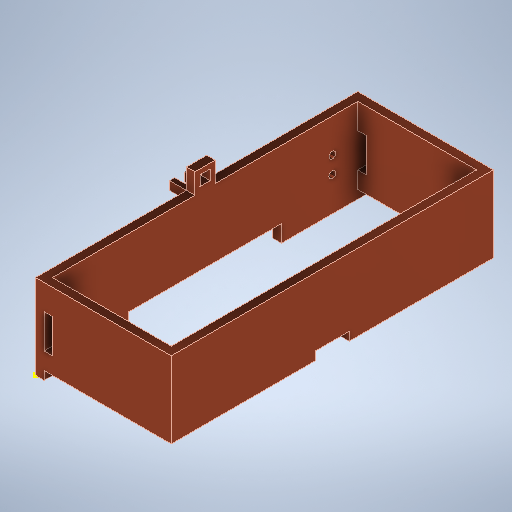
# Autodesk Inventor part: cover
Saved by Autodesk Inventor 2025.3 (Build 293356030, 356C)
## iProperties
Created: 2026-06-26
Part Number: cover
Material: Generic
Document SubType Name: Modeling
Designer: user
Density: 1 g/cm^3
Appearance: Copper - Polished
Author: user
Autodesk Inventor part; units mm, degrees
ref_plane "YZ Plane" through (0, 0, 0) normal (1, 0, 0) x (0, 1, 0)
ref_plane "XZ Plane" through (0, 0, 0) normal (0, 1, 0) x (-1, 0, 0)
ref_plane "XY Plane" through (0, 0, 0) normal (0, 0, 1) x (1, 0, 0)
sketch "Sketch1" plane through (0, 0, 0) normal (1, 0, 0) x (0, 1, 0)
  line L0 (0, 0) -> (50, 0)
  line L1 (50, 0) -> (50, -50)
  line L2 (0, 0) -> (10, 0)
  line L3 (10, -50) -> (0, -50)
  line L4 (0, -50) -> (0, 0)
  line L5 (50, -50) -> (50, -190)
  line L6 (50, -190) -> (0, -190)
  line L7 (0, -190) -> (0, -140)
  line L8 (0, -140) -> (10, -140)
  line L9 (10, -140) -> (10, -50)
  line L10 (0, -105) -> (50, -105) construction
  line L11 (50, -89) -> (62, -89)
  line L12 (62, -89) -> (62, -101)
  line L13 (62, -101) -> (50, -101)
  line L14 (50, -101) -> (50, -89)
  line L15 (59, -92) -> (53, -92)
  line L16 (53, -92) -> (53, -98)
  line L17 (53, -98) -> (59, -98)
  line L18 (59, -98) -> (59, -92)
  point P0 (50, -101)
  dimension "d0" = 50
  dimension "d4" = 50
  dimension "d5" = 10
  dimension "d8" = 190
  dimension "d9" = 50
  dimension "d10" = 12
  dimension "d11" = 12
  dimension "d12" = 3
  dimension "d19" = 89
  constraints: 38 end point, 8 perpendicular, 5 parallel, 3 horizontal, 2 point on line, 1 vertical, 3 other
  measures "d0" distance of L0.start L0.end
  measures "d4" distance of L6.end L7.end
  measures "d5" distance of L7.end L8.end
  measures "d8" distance between parallel lines of L0 L6
  measures "d9" distance of L3.end L0.start
  measures "d10" distance of L12.end L13.end
  measures "d11" distance of L11.end L12.end
  measures "d12" distance between parallel lines of L11 L15
  measures "d19" distance between parallel lines of L0 L11
extrude "Extrusion1" add sketch "Sketch1" along normal blind 5
sketch "Sketch2" plane through (0, 0, 0) normal (-1, 0, 0) x (0, 0, 1)
  line L0 (-190, 50) -> (-101, 50) projected
  line L1 (-101, 50) -> (-89, 50)
  line L2 (-89, 50) -> (-89, 45)
  line L3 (-89, 45) -> (-101, 45)
  line L4 (-101, 45) -> (-101, 50)
  point P0 (0, 0)
  dimension "d13" = 5
  constraints: 8 end point, 2 parallel, 1 horizontal, 1 perpendicular
  measures "d13" distance of L1.end L2.end
extrude "Extrusion2" add sketch "Sketch2" along normal blind 10
sketch "Sketch3" plane through (0, 50, -89) normal (0, 1, 0) x (1, 0, 0)
  line L0 (-10, 12) -> (-10, 0) projected
  line L1 (0, 0) -> (0, 12) projected
  line L2 (-10, 3) -> (0, 3)
  line L3 (0, 3) -> (0, 9)
  line L4 (0, 9) -> (-10, 9)
  line L5 (-10, 9) -> (-10, 3)
  point P0 (0, -89)
  point P1 (-10, 9)
  point P2 (0, 3)
  dimension "d16" = 6
  constraints: 8 end point, 2 parallel, 2 point on line, 1 horizontal, 1 perpendicular
  measures "d16" distance of L3.end L2.end
extrude "Extrusion3" cut sketch "Sketch3" against normal blind 10
sketch "Sketch4" plane through (5, 0, 0) normal (1, 0, 0) x (0, 0, -1)
  line L0 (89, 50) -> (0, 50) projected
  line L1 (0, 0) -> (50, 0) projected
  line L2 (190, 50) -> (101, 50) projected
  line L3 (0, 50) -> (5, 50)
  line L4 (5, 50) -> (5, 5)
  line L5 (5, 5) -> (0, 5)
  line L6 (0, 5) -> (0, 50)
  line L7 (190, 0) -> (190, 50) projected
  line L8 (185, 50) -> (190, 50)
  line L9 (190, 50) -> (190, 5)
  line L10 (190, 5) -> (185, 5)
  line L11 (185, 5) -> (185, 50)
  point P0 (5, 0)
  dimension "d27" = 5
  dimension "d28" = 45
  dimension "d32" = 45
  constraints: 16 end point, 4 parallel, 3 point on line, 2 horizontal, 2 perpendicular
  measures "d27" distance of L4.end L5.end
  measures "d28" distance of L3.end L4.end
  measures "d32" distance of L10.end L8.start
extrude "Extrusion4" add sketch "Sketch4" along normal blind 75
sketch "Sketch6" plane through (0, 0, 0) normal (0, 0, 1) x (1, 0, 0)
  point P0 (0, 0)
sketch "Sketch7" plane through (5, 5, -185) normal (0, 0, 1) x (1, 0, 0)
  line L0 (0, 45) -> (75, 45) projected
  line L1 (0, 0) -> (75, 0) projected
  line L2 (75, 45) -> (70, 45)
  line L3 (70, 45) -> (70, 0)
  line L4 (70, 0) -> (75, 0)
  line L5 (75, 0) -> (75, 45)
  point P0 (-5, -5)
  dimension "d29" = 5
  constraints: 8 end point, 2 parallel, 1 horizontal, 1 perpendicular, 1 point on line
  measures "d29" distance of L4.end L3.end
extrude "Extrusion6" add sketch "Sketch7" along normal blind 180
sketch "Sketch8" plane through (80, 0, 0) normal (1, 0, 0) x (0, 0, -1)
  line L0 (50, 10) -> (140, 10) projected
  line L1 (85, 5) -> (105, 5)
  line L2 (105, 5) -> (105, 10)
  line L3 (105, 10) -> (85, 10)
  line L4 (85, 10) -> (85, 5)
  point P0 (0, 0)
  dimension "d33" = 20
  constraints: 8 end point, 2 parallel, 1 horizontal, 1 perpendicular, 1 point on line
  measures "d33" distance of L3.end L2.end
extrude "Extrusion7" cut sketch "Sketch8" against normal blind 180
sketch "Sketch9" plane through (5, 0, 0) normal (1, 0, 0) x (0, 0, -1)
  circle A0 centre (20, 30) radius 2
  circle A1 centre (20, 20) radius 2
  circle A2 centre (170, 30) radius 2
  circle A3 centre (170, 20) radius 2
  line L0 (0, 50) -> (0, 5) projected
  line L1 (190, 5) -> (190, 50) projected
  line L2 (89, 50) -> (5, 50) projected
  line L3 (185, 50) -> (101, 50) projected
  point P0 (0, 0)
  dimension "d36" = 4
  dimension "d37" = 4
  dimension "d38" = 4
  dimension "d39" = 4
  dimension "d40" = 20
  dimension "d41" = 20
  dimension "d42" = 20
  dimension "d43" = 20
  dimension "d44" = 10
  dimension "d45" = 10
  dimension "d46" = 20
  dimension "d47" = 20
  constraints: 4 centre point
  measures "d36" diameter of A0
  measures "d37" diameter of A1
  measures "d38" diameter of A2
  measures "d39" diameter of A3
  measures "d40" distance from line of A0.centre L0
  measures "d41" distance from line of L0 A1.centre
  measures "d42" distance from line of L1 A2.centre
  measures "d43" distance from line of L1 A3.centre
  measures "d44" distance of A3.centre A2.centre
  measures "d45" distance of A1.centre A0.centre
  measures "d46" distance from line of L2 A0.centre
  measures "d47" distance from line of L3 A2.centre
extrude "Extrusion8" cut sketch "Sketch9" against normal blind 180
sketch "Sketch10" plane through (0, 0, -190) normal (0, 0, -1) x (-1, 0, 0)
  line L0 (-5, 50) -> (-5, 5) projected
  line L1 (-5, 15) -> (-10, 15)
  line L2 (-10, 15) -> (-10, 35)
  line L3 (-10, 35) -> (-5, 35)
  line L4 (-5, 35) -> (-5, 15)
  point P0 (0, 0)
  dimension "d50" = 5
  dimension "d51" = 20
  constraints: 8 end point, 2 parallel, 1 horizontal, 1 perpendicular, 1 point on line
  measures "d50" distance of L2.end L3.end
  measures "d51" distance of L1.end L2.end
extrude "Extrusion9" cut sketch "Sketch10" against normal through all
body "Solid1"
